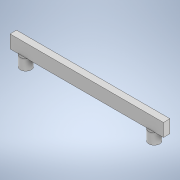
# Autodesk Inventor part: dsadas
Saved by Autodesk Inventor 2020 (Build 240168000, 168)
## iProperties
Created: 2021-12-16
Part Number: dsadas
Material: Generic
Document SubType Name: Modeling
Designer: FadyR
Density: 1 g/cm^3
Appearance: Default
Author: FadyR
Autodesk Inventor part; units mm, degrees
ref_plane "YZ Plane" through (0, 0, 0) normal (1, 0, 0) x (0, 1, 0)
ref_plane "XZ Plane" through (0, 0, 0) normal (0, 1, 0) x (-1, 0, 0)
ref_plane "XY Plane" through (0, 0, 0) normal (0, 0, 1) x (1, 0, 0)
sketch "Sketch1" plane through (0, 0, 0) normal (0, 1, 0) x (-1, 0, 0)
  point P0 (0, 0)
sketch "Sketch2" plane through (0, 0, 0) normal (0, 1, 0) x (-1, 0, 0)
  line L0 (30, -1.27) -> (-30, -1.27)
  line L1 (-30, -1.27) -> (-30, 1.27)
  line L2 (-30, 1.27) -> (30, 1.27)
  line L3 (30, 1.27) -> (30, -1.27)
  line L4 (30, -1.27) -> (-30, 1.27) construction
  line L5 (-30, -1.27) -> (30, 1.27) construction
  point P0 (0, 0)
  dimension "d0" = 60
  dimension "d1" = 2.54
  constraints: 12 end point, 2 midpoint, 2 parallel, 1 horizontal, 1 perpendicular
  measures "d0" distance of L1.end L2.end
  measures "d1" distance of L0.end L1.end
extrude "Extrusion1" add sketch "Sketch2" along normal blind 5.08
sketch "Sketch3" plane through (0, 0, 0) normal (0, -1, 0) x (1, 0, 0)
  circle A0 centre (-25.1, 0) radius 2.15
  line L0 (-30, -1.27) -> (-30, 1.27) projected
  circle A1 centre (25.1, 0) radius 2.15
  line L1 (30, 1.27) -> (30, -1.27) projected
  point P0 (0, 0)
  dimension "d4" = 4.3
  dimension "d5" = 4.9
  dimension "d6" = 4.3
  dimension "d7" = 4.9
  constraints: 2 centre point
  measures "d4" diameter of A0
  measures "d5" distance from line of L0 A0.centre
  measures "d6" diameter of A1
  measures "d7" distance from line of L1 A1.centre
extrude "Extrusion2" add sketch "Sketch3" along normal blind 4.2
body "Solid1"
